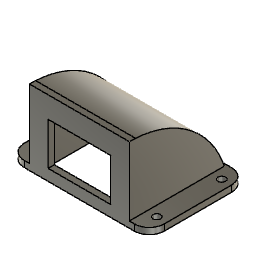
Sem título (Autodesk Fusion 360 design; units mm, degrees)
Autodesk Fusion 360 part; units mm, degrees
note: some values were not read from the file. Chosen so that the rebuilt part matches the saved one: that a step has no effect.
sketch "Esboço1" plane through (0, 0, 0) normal (0, 0, 1) x (1, 0, 0)
  line L0 (20, 20) -> (-20, 20)
  line L1 (-20, 20) -> (-20, -20)
  line L2 (-20, -20) -> (20, -20)
  line L3 (20, -20) -> (20, 20)
  line L4 (20, 20) -> (-20, -20) construction
  line L5 (-20, 20) -> (20, -20) construction
  line L6 (-17.5, -17.5) -> (17.5, -17.5)
  line L7 (17.5, -17.5) -> (17.5, 17.5)
  line L8 (17.5, 17.5) -> (-17.5, 17.5)
  line L9 (-17.5, 17.5) -> (-17.5, -17.5)
  dimension "d1" = 40
  dimension "d2" = 40
  dimension "d3" = -2.5
  constraint horizontal L0
  constraint perpendicular L0 L1
  constraint parallel L0 L2
  constraint parallel L1 L3
  constraint coincident L4 origin
  constraint coincident L5 origin
  measures "d1" distance of L1.end L2.end
  measures "d2" distance of L0.end L1.end
extrude "Extrusão1" add sketch "Esboço1" along normal blind 30
sketch "Esboço2" plane through (20, 0, 0) normal (1, 0, 0) x (0, 1, 0)
  line L0 (-20, 0) -> (20, 0)
  line L1 (20, 0) -> (20, 30)
  line L2 (20, 30) -> (-20, 30)
  line L3 (-20, 30) -> (-20, 0)
  line L4 (-20, 0) -> (20, 0)
  line L5 (20, 0) -> (20, -10)
  line L6 (-20, 30) -> (-20, 0)
  arc A0 (20, -10) -> (-20, 30) centre (-20, -10) ccw
  line L7 (-17.5, 2.5) -> (15.3553, 2.5)
  arc A1 (15.3553, 2.5) -> (-17.5, 27.4166) centre (-20, -10) ccw
  line L8 (-17.5, 27.4166) -> (-17.5, 2.5)
  line L9 (-17.5, 27.4166) -> (-20, 27.5836)
  line L10 (15.3553, 2.5) -> (16.2392, 0)
  dimension "d7" = 40
  dimension "d8" = -2.5
  constraint tangent L5 A0
  constraint coincident L2.end L3.start
  constraint coincident L6 L9.end
  constraint tangent A1 L9
  constraint coincident L4 L10.end
  constraint tangent A1 L10
  measures "d7" radius of A0
extrude "Extrusão2" add sketch "Esboço2" against normal blind 57.5 contours L0 L3 L4 L6 A0 A1 L9 L10
sketch "Esboço3" plane through (17.5, 0, 0) normal (-1, 0, 0) x (0, -1, 0)
  arc A0 (17.5, 29.9218) -> (-17.5, 3.9194) centre (20, -10) ccw
  line L0 (17.5, 29.9218) -> (17.5, 30)
  line L1 (17.5, 30) -> (-17.5, 30)
  line L2 (-17.5, 30) -> (-17.5, 3.9194)
  line L3 (20, 30) -> (24, 38)
  line L4 (24, 38) -> (-25, 34)
  line L5 (-25, 34) -> (-26, 0)
  line L6 (-26, 0) -> (-20, 0)
  arc A1 (17.5, 29.9218) -> (-17.5, 3.9194) centre (20, -10) ccw
  line L7 (17.5, 29.9218) -> (20, 30)
  line L8 (-17.5, 3.9194) -> (-20, 0)
  line L9 (-17.5, 3.9194) -> (-17.5931, 3.6686)
  line L10 (-17.5931, 3.6686) -> (-18.9548, 0)
  line L11 (-20, 0) -> (-18.9548, 0)
  dimension "d11" = 0
  constraint parallel L1 L6
  constraint tangent A1 L9
  constraint parallel L9 L10
  constraint parallel L6 L11
extrude "Extrusão3" cut sketch "Esboço3" along normal blind 70 and the other way blind 20
sketch "Esboço4" plane through (0, 0, 0) normal (0, 0, -1) x (1, 0, 0)
  line L0 (-20, -18.9548) -> (20, -18.9548)
  line L1 (20, -18.9548) -> (20, 20)
  line L2 (20, 20) -> (-20, 20)
  line L3 (-20, 20) -> (-20, -16.2392)
  line L4 (-20, -16.2392) -> (-37.5, -16.2392)
  line L5 (-17.5, -16.2392) -> (-17.5, 17.5)
  line L6 (-17.5, 17.5) -> (17.5, 17.5)
  line L7 (17.5, 17.5) -> (17.5, -16.2392)
  line L8 (-20, -18.9548) -> (-35, -18.9548)
  line L9 (-40, -13.9548) -> (-40, 15)
  line L10 (-35, 20) -> (-20, 20)
  line L11 (-20, 20) -> (-20, -18.9548)
  line L12 (0, 0) -> (0, -7)
  line L13 (20, 20) -> (20, -18.9548)
  line L14 (20, -18.9548) -> (35, -18.9548)
  line L15 (40, -13.9548) -> (40, 15)
  line L16 (35, 20) -> (20, 20)
  line L17 (-35, 20) -> (-35, 12)
  circle A0 centre (-35, 12) radius 1.5
  line L18 (-40, 0) -> (-43, 0)
  circle A1 centre (-35, -12) radius 1.5
  circle A2 centre (35, -12) radius 1.5
  circle A3 centre (35, 12) radius 1.5
  arc A4 (35, -18.9548) -> (40, -13.9548) centre (35, -13.9548) ccw
  arc A5 (40, 15) -> (35, 20) centre (35, 15) ccw
  arc A6 (-40, -13.9548) -> (-35, -18.9548) centre (-35, -13.9548) ccw
  arc A7 (-35, 20) -> (-40, 15) centre (-35, 15) ccw
  line L19 (-37.5, -16.2392) -> (-37.5, -18.7298)
  line L20 (-37.5, -18.7298) -> (-20, -18.7298)
  line L21 (-20, -18.7298) -> (-20, -18.9548)
  line L22 (17.5, -16.2392) -> (-17.5, -16.2392)
  dimension "d16" = 8
  dimension "d17" = 3
  dimension "d18" = 5
  constraint horizontal L8
  constraint vertical L9
  constraint horizontal L10
  constraint vertical L11
  constraint coincident L0.start L8.start
  constraint coincident L12.start origin
  constraint vertical L12
  constraint symmetric L0.start L12 L0.end
  constraint symmetric L2.end L12 L1.end
  constraint perpendicular L10 L17
  constraint coincident L17.end A0.centre
  constraint coincident L9 L18.start
  constraint perpendicular L9 L18
  constraint symmetric A0 L18 A1
  constraint symmetric L12 A0 A3
  constraint symmetric L12 A1 A2
  constraint tangent L15 A4
  constraint tangent L14 A4
  constraint tangent L15 A5
  constraint tangent L16 A5
  constraint equal A4 A5
  constraint tangent L8 A6
  constraint tangent L9 A6
  constraint equal A4 A6
  constraint coincident L10 L17.start
  constraint tangent L9 A7
  constraint tangent L10 A7
  constraint equal A4 A7
  measures "d16" distance of L10.start L17.end
  measures "d17" diameter of A0
  measures "d18" radius of A4
extrude "Extrusão4" add sketch "Esboço4" against normal blind 2.5 contours L8 L11 A6 L20 L21 | L1 L13 L14 L15 L16 A4 A5 | L4 L11 A6 L19 L20 | L3 L4 L9 L10 L11 A6 A7 L19
chamfer "Chanfro1" [no effect]
extrude "Extrusão5" add 1 faces at (-20, 18.6455, 1.6667) along direction (1, 0, 0) blind 60
sketch "Esboço5" plane through (0, -20, 0) normal (0, -1, 0) x (1, 0, 0)
  line L0 (-35, 0) -> (35, 0)
  line L1 (35, 0) -> (35, 2.5)
  line L2 (35, 2.5) -> (20, 2.5)
  line L3 (20, 2.5) -> (20, 30)
  line L4 (20, 30) -> (-37.5, 30)
  line L5 (-37.5, 30) -> (-37.5, 27.5836)
  line L6 (-37.5, 27.5836) -> (-20, 27.5836)
  line L7 (-20, 27.5836) -> (-20, 2.5)
  line L8 (-20, 2.5) -> (-35, 2.5)
  line L9 (-35, 2.5) -> (-35, 0)
  line L10 (-20, 2.5) -> (-45, 2.5)
  line L11 (-45, 2.5) -> (-45, 38)
  line L12 (-45, 38) -> (-20, 38)
  line L13 (-20, 38) -> (-20, 2.5)
  constraint horizontal L10
  constraint vertical L11
  constraint horizontal L12
  constraint vertical L13
  constraint coincident L7.end L8.start
extrude "Extrusão6" cut sketch "Esboço5" against normal blind 45 contours L4 L5 L6 L7 L8 L10 L11 L12 L13 | L4 L5 L6 L13
sketch "Esboço6" plane through (0, 0, 0) normal (0, 0, -1) x (1, 0, 0)
  circle A0 centre (35, 12) radius 1.5
  circle A1 centre (35, -12) radius 1.5
  circle A2 centre (-35, -12) radius 1.5
  circle A3 centre (-35, 12) radius 1.5
  line L0 (17.5, -16.2392) -> (-17.5, -16.2392)
  line L1 (-17.5, -16.2392) -> (-17.5, 17.5)
  line L2 (-17.5, 17.5) -> (17.5, 17.5)
  line L3 (17.5, 17.5) -> (17.5, -16.2392)
  line L4 (-37.5, -18.285) -> (-37.5, -18.7298)
  line L5 (-37.5, -18.7298) -> (-36.483, -18.7298)
  arc A4 (-36.483, -18.7298) -> (-35, -18.9548) centre (-35, -13.9548) ccw
  line L6 (-35, -18.9548) -> (35, -18.9548)
  arc A5 (35, -18.9548) -> (40, -13.9548) centre (35, -13.9548) ccw
  line L7 (40, -13.9548) -> (40, 15)
  arc A6 (40, 15) -> (35, 20) centre (35, 15) ccw
  line L8 (35, 20) -> (-35, 20)
  arc A7 (-35, 20) -> (-40, 15) centre (-35, 15) ccw
  line L9 (-40, 15) -> (-40, -13.9548)
  arc A8 (-40, -13.9548) -> (-37.5, -18.285) centre (-35, -13.9548) ccw
  line L10 (28, 20) -> (-28, 20)
  line L11 (-28, 20) -> (-28, -20)
  line L12 (-28, -20) -> (28, -20)
  line L13 (28, -20) -> (28, 20)
  line L14 (28, 20) -> (-28, -20) construction
  line L15 (-28, 20) -> (28, -20) construction
  line L16 (28, 20) -> (46, 22)
  line L17 (46, 22) -> (45, -23)
  line L18 (45, -23) -> (-45, -25)
  line L19 (-45, -25) -> (-43.9778, 21)
  line L20 (-43.9778, 21) -> (-28, 24)
  line L21 (-28, 24) -> (-28, 20)
  constraint horizontal L10
  constraint perpendicular L10 L11
  constraint parallel L10 L12
  constraint parallel L11 L13
  constraint coincident L14 origin
  constraint coincident L15 origin
  constraint coincident L8 L10.start
  constraint parallel L17 L19
  constraint perpendicular L8 L21
extrude "Extrusão7" cut sketch "Esboço6" against normal blind 10 contours L4 L5 A4 L6 L8 A7 L9 A8 L11 | L4 L5 A4 L6 A5 L7 A6 L8 A7 L9 A8 L11 L12 L13 L16 L17 L18 L19 L20 L21 | L6 A5 L7 A6 L8 L13
sketch "Esboço7" plane through (0, 0, 0) normal (0, 0, -1) x (1, 0, 0)
  line L0 (28, -18.9548) -> (28, 20)
  line L1 (28, 20) -> (-28, 20)
  line L2 (-28, 20) -> (-28, -18.9548)
  line L3 (-28, -18.9548) -> (28, -18.9548)
  line L4 (17.5, -16.2392) -> (-17.5, -16.2392)
  line L5 (-17.5, -16.2392) -> (-17.5, 17.5)
  line L6 (-17.5, 17.5) -> (17.5, 17.5)
  line L7 (17.5, 17.5) -> (17.5, -16.2392)
  line L8 (-28, 20) -> (-24, 20)
  line L9 (-24, 20) -> (-24, 13)
  circle A0 centre (-24, 13) radius 1.5
  line L10 (-28, 0) -> (-25, 0)
  line L11 (0, 0) -> (0, 5.5291)
  circle A1 centre (-24, -13) radius 1.5
  circle A2 centre (24, 13) radius 1.5
  circle A3 centre (24, -13) radius 1.5
  dimension "d28" = 4
  dimension "d29" = 7
  dimension "d30" = 3
  constraint coincident L1.end L2.start
  constraint perpendicular L2 L8
  constraint perpendicular L1 L9
  constraint coincident L9.end A0.centre
  constraint coincident L2 L10.start
  constraint perpendicular L2 L10
  constraint coincident L11.start origin
  constraint vertical L11
  constraint symmetric A0 L10 A1
  constraint symmetric A0 L11 A2
  constraint symmetric L11 A1 A3
  measures "d28" distance of L1.end L8.end
  measures "d29" distance of L8.end L9.end
  measures "d30" diameter of A0
extrude "Extrusão8" cut sketch "Esboço7" against normal blind 6 contours A0 | A1 | A2 | A3
sketch "Esboço8" plane through (0, 0, 0) normal (0, 0, -1) x (1, 0, 0)
  circle A0 centre (24, -13) radius 1.5
  circle A1 centre (-24, -13) radius 1.5
  circle A2 centre (24, 13) radius 1.5
  circle A3 centre (-24, 13) radius 1.5
  line L0 (28, -18.9548) -> (28, 20)
  line L1 (28, 20) -> (-28, 20)
  line L2 (-28, 20) -> (-28, -18.9548)
  line L3 (-28, -18.9548) -> (28, -18.9548)
  line L4 (17.5, -16.2392) -> (-17.5, -16.2392)
  line L5 (-17.5, -16.2392) -> (-17.5, 17.5)
  line L6 (-17.5, 17.5) -> (17.5, 17.5)
  line L7 (17.5, 17.5) -> (17.5, -16.2392)
  line L8 (-22, -18.9548) -> (22, -18.9548)
  line L9 (28, -12.9548) -> (28, 14)
  line L10 (22, 20) -> (-22, 20)
  line L11 (-28, 14) -> (-28, -12.9548)
  arc A4 (-22, 20) -> (-28, 14) centre (-22, 14) ccw
  arc A5 (28, 14) -> (22, 20) centre (22, 14) ccw
  arc A6 (22, -18.9548) -> (28, -12.9548) centre (22, -12.9548) ccw
  arc A7 (-28, -12.9548) -> (-22, -18.9548) centre (-22, -12.9548) ccw
  dimension "d34" = 6
  constraint tangent L11 A4
  constraint tangent L10 A4
  constraint tangent L10 A5
  constraint tangent L9 A5
  constraint equal A4 A5
  constraint tangent L9 A6
  constraint tangent L8 A6
  constraint equal A4 A6
  constraint tangent L11 A7
  constraint tangent L8 A7
  constraint equal A4 A7
  measures "d34" radius of A4
extrude "Extrusão9" cut sketch "Esboço8" against normal blind 3 contours L0 L3 A6 | L0 L1 A5 | L2 L3 A7 | L1 L2 A4
sketch "Esboço9" plane through (0, -20, 0) normal (0, -1, 0) x (1, 0, 0)
  line L0 (-22, 2.5) -> (-22, 0)
  line L1 (-22, 0) -> (22, 0)
  line L2 (22, 0) -> (22, 2.5)
  line L3 (22, 2.5) -> (20, 2.5)
  line L4 (20, 2.5) -> (20, 30)
  line L5 (20, 30) -> (-20, 30)
  line L6 (-20, 30) -> (-20, 2.5)
  line L7 (-20, 2.5) -> (-22, 2.5)
  line L8 (-17.5, 2.5) -> (17.5, 2.5)
  line L9 (17.5, 2.5) -> (17.5, 27.5)
  line L10 (17.5, 27.5) -> (-17.5, 27.5)
  line L11 (-17.5, 27.5) -> (-17.5, 2.5)
  line L12 (0, 27.5) -> (0, 21.5)
  line L13 (0, 21.5) -> (0, 4.5) construction
  line L14 (12.5, 4.5) -> (-12.5, 4.5)
  line L15 (-12.5, 4.5) -> (-12.5, 21.5)
  line L16 (-12.5, 21.5) -> (12.5, 21.5)
  line L17 (12.5, 21.5) -> (12.5, 4.5)
  line L18 (12.5, 4.5) -> (-12.5, 21.5) construction
  line L19 (-12.5, 4.5) -> (12.5, 21.5) construction
  point P0 (0, 13)
  dimension "d37" = -2.5
  dimension "d38" = 6
  dimension "d39" = 17
  dimension "d40" = 25
  constraint midpoint L10 L12.start
  constraint perpendicular L10 L12
  constraint perpendicular L10 L13
  constraint horizontal L14
  constraint perpendicular L14 L15
  constraint parallel L14 L16
  constraint parallel L15 L17
  constraint coincident L18 P0
  constraint coincident L19 P0
  constraint midpoint L13 P0
  measures "d38" distance of L12.start L12.end
  measures "d39" distance of L12.end L13.end
  measures "d40" distance of L15.end L16.end
extrude "Extrusão10" cut sketch "Esboço9" against normal blind 3 contours L14 L15 L16 L17
